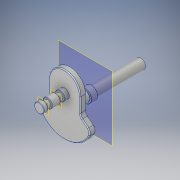
# Autodesk Inventor part: piston rod
Saved by Autodesk Inventor 2018 (Build 220112000, 112)
## iProperties
Created: 2018-02-21
Part Number: piston rod
Material: Aluminum 6061
Document SubType Name: Modeling
Designer: 238438
Density: 2.7 g/cm^3
Appearance: Aluminum - Flat
Author: 238438
Autodesk Inventor part; units mm, degrees
ref_plane "YZ Plane" through (0, 0, 0) normal (1, 0, 0) x (0, 1, 0)
ref_plane "XZ Plane" through (0, 0, 0) normal (0, 1, 0) x (-1, 0, 0)
ref_plane "XY Plane" through (0, 0, 0) normal (0, 0, 1) x (1, 0, 0)
sketch "Sketch1" plane through (0, 0, 0) normal (0, 0, 1) x (1, 0, 0)
  arc A0 (-8.0545, -2.54) -> (8.0545, -2.54) centre (0, 0) ccw
  line L0 (-8.0545, -2.54) -> (-4.8148, 0.1784)
  line L1 (8.0545, -2.54) -> (4.8148, 0.1784)
  line L2 (-4.8148, 0.1784) -> (-4.8148, 5.2584)
  line L3 (4.8148, 0.1784) -> (4.8148, 5.2584)
  arc A1 (4.8148, 5.2584) -> (-4.8148, 5.2584) centre (0, 5.2584) ccw
  line L4 (-4.8148, 5.2584) -> (-4.8148, 0.1784)
  line L5 (-4.8148, 0.1784) -> (-8.0545, -2.54)
  line L6 (4.8148, 0.1784) -> (8.0545, -2.54)
  line L7 (4.8148, 0.1784) -> (4.8148, 5.2584)
  arc A2 (4.8148, 5.2584) -> (-4.8148, 5.2584) centre (0, 5.2584) ccw
  arc A3 (-8.0545, -2.54) -> (8.0545, -2.54) centre (0, 0) ccw
  dimension "d6" = 5.08
  dimension "d7" = 5.08
  constraints: 16 end point, 8 point on circle, 4 centre point, 3 vertical, 2 collinear, 2 tangent
  measures "d6" distance of L0.end L2.end
  measures "d7" distance of L3.start L3.end
extrude "Extrusion1" add sketch "Sketch1" along normal blind 1.8542
fillet "Fillet1" radius 1.5875 4 edges at (8.0545, -2.54, 0.9271) (-8.0545, -2.54, 0.9271) (-4.8148, 0.1784, 0.9271) (4.8148, 0.1784, 0.9271)
fillet "Fillet2" radius 0.254 20 edges at (-4.8148, 3.0885, 1.8542) (-4.9636, 0.2478, 1.8542) (-6.2797, -1.0508, 1.8542) (-7.7103, -2.6919, 1.8542) (0, -8.4455, 1.8542) (7.7103, -2.6919, 1.8542) (6.2797, -1.0508, 1.8542) (4.9636, 0.2478, 1.8542) (4.8148, 3.0885, 1.8542) (0, 10.0732, 1.8542) (-4.8148, 3.0885, 0) (-4.9636, 0.2478, 0) (-6.2797, -1.0508, 0) (-7.7103, -2.6919, 0) (0, -8.4455, 0) (7.7103, -2.6919, 0) (6.2797, -1.0508, 0) (4.9636, 0.2478, 0) (4.8148, 3.0885, 0) (0, 10.0732, 0)
sketch "Sketch2" plane through (0, 0, 1.8542) normal (0, 0, 1) x (1, 0, 0)
  line L0 (4.5608, 5.2584) -> (4.8148, 5.2584) projected
  line L1 (-4.8148, 5.2584) -> (-4.8148, 0.9187) projected
  arc A0 (4.5608, 5.2584) -> (-4.5608, 5.2584) centre (0, 5.2584) ccw projected
  circle A1 centre (0, 3.7852) radius 1.4732
  circle A2 centre (0, 3.7852) radius 1.4732
  point P0 (0, 0)
  constraints: 2 centre point, 1 coincident, 1 concentric
extrude "Extrusion2" add sketch "Sketch2" along normal blind 7.7597
ref_plane "Work Plane1" through (0, 3.7852, 8.3439) normal (0, 0, 1) x (1, 0, 0)
sketch "Sketch3" plane through (0, 3.7852, 8.3439) normal (0, 0, 1) x (1, 0, 0)
  circle A0 centre (0, 0) radius 0.9906
  circle A1 centre (0, 0) radius 1.4732
  point P0 (0, -3.7852)
  dimension "d18" = 1.9812
  constraints: 2 centre point, 1 coincident
  measures "d18" diameter of A0
extrude "Extrusion3" cut sketch "Sketch3" against normal blind 1.27
ref_plane "Work Plane2" through (0, 3.7852, 4.5339) normal (0, 0, 1) x (1, 0, 0)
sketch "Sketch4" plane through (0, 3.7852, 4.5339) normal (0, 0, 1) x (1, 0, 0)
  circle A0 centre (0, 0) radius 0.9906
  circle A1 centre (0, 0) radius 1.4732
  point P0 (0, -3.7852)
  constraints: 2 centre point, 1 coincident
extrude "Extrusion4" cut sketch "Sketch4" against normal blind 1.27
chamfer "Chamfer1" distance 0.127 angle 45 5 edges at (-1.4732, 3.7852, 9.6139) (-1.4732, 3.7852, 8.3439) (-1.4732, 3.7852, 7.0739) (-1.4732, 3.7852, 4.5339) (-1.4732, 3.7852, 3.2639)
sketch "Sketch5" plane through (0, 0, 1.8542) normal (0, 0, 1) x (1, 0, 0)
  circle A0 centre (0, 0) radius 1.4668
  dimension "d27" = 2.9337
  constraints: 1 centre point, 1 coincident
  measures "d27" diameter of A0
extrude "Extrusion5" add sketch "Sketch5" against normal blind 23.368
sketch "Sketch6" plane through (0, 0, -21.5138) normal (0, 0, -1) x (-1, 0, 0)
  point P0 (0, 0)
  point P1 (0, 0)
  constraints: 1 coincident
hole "Hole1" at (0, 0, -21.5138) direction (0, 0, 1) diameter 1.905 depth 4.0132 tip angle 118 countersink diameter 2.54 countersink angle 45
thread "Thread1" size "1-64 UNC" class "2B" standard "ANSI Unified Screw Threads" full length
ref_plane "Work Plane3" through (0, 0, -4.445) normal (0, 0, -1) x (-1, 0, 0)
sketch "Sketch7" plane through (0, 0, -4.445) normal (0, 0, -1) x (-1, 0, 0)
  circle A0 centre (0, 0) radius 1.4668
  circle A1 centre (0, 0) radius 1.9748
  dimension "d40" = 3.9497
  constraints: 2 centre point, 2 coincident
  measures "d40" diameter of A1
extrude "Extrusion6" add sketch "Sketch7" along normal blind 1.905
fillet "Fillet3" radius 0.0635 2 edges at (1.9748, 0, -6.35) (1.9748, 0, -4.445)
fillet "Fillet4" radius 0.0635 2 edges at (-1.4668, 0, -6.35) (-1.4668, 0, -4.445)
body "Solid1"
